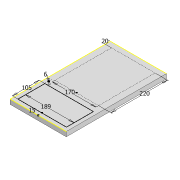
# Autodesk Inventor part: Platform
Saved by Autodesk Inventor 2020 (Build 240168000, 168)
## iProperties
Created: 2021-06-25
Part Number: Platform
Material: Generic
Document SubType Name: Modeling
Designer: Aidan Lee
Density: 1 g/cm^3
Appearance: Default
Author: Aidan Lee
Autodesk Inventor part; units mm, degrees
ref_plane "YZ Plane" through (0, 0, 0) normal (1, 0, 0) x (0, 1, 0)
ref_plane "XZ Plane" through (0, 0, 0) normal (0, 1, 0) x (-1, 0, 0)
ref_plane "XY Plane" through (0, 0, 0) normal (0, 0, 1) x (1, 0, 0)
sketch "Sketch1" plane through (0, 0, 0) normal (0, 0, 1) x (1, 0, 0)
  line L0 (0, 0) -> (219, 0)
  line L1 (219, 0) -> (219, 18)
  line L2 (219, 18) -> (0, 18)
  line L3 (0, 18) -> (0, 0)
  dimension "d0" = 18
  dimension "d1" = 219
  constraints: 8 end point, 2 parallel, 1 horizontal, 1 perpendicular
  measures "d0" distance of L2.end L0.start
  measures "d1" distance of L0.start L0.end
extrude "Extrusion1" add sketch "Sketch1" against normal blind 390
sketch "Sketch2" plane through (0, 18, 0) normal (0, 1, 0) x (1, 0, 0)
  line L0 (24.5, 150) -> (194.5, 150) construction
  line L1 (194.5, 150) -> (194.5, 370) construction
  line L2 (194.5, 370) -> (24.5, 370) construction
  line L3 (24.5, 370) -> (24.5, 150) construction
  line L4 (15, 15) -> (204, 15)
  line L5 (204, 15) -> (204, 120)
  line L6 (204, 120) -> (15, 120)
  line L7 (15, 120) -> (15, 15)
  line L8 (219, 0) -> (0, 0) projected
  line L9 (0, 0) -> (0, 390) projected
  line L10 (0, 390) -> (219, 390) projected
  circle A0 centre (15, 135) radius 3
  line L11 (15, 120) -> (15, 150) construction
  point P0 (109.5, 0)
  point P1 (109.5, 15)
  point P2 (109.5, 0)
  point P3 (109.5, 150)
  point P4 (15, 135)
  dimension "d4" = 220
  dimension "d5" = 170
  dimension "d6" = 189
  dimension "d7" = 105
  dimension "d9" = 15
  dimension "d11" = 20
  dimension "d12" = 6
  constraints: 18 end point, 5 midpoint, 4 parallel, 3 vertical alignment, 2 horizontal, 2 perpendicular, 1 centre point, 1 coincident, 1 horizontal alignment, 1 vertical
  measures "d4" distance of L0.end L1.end
  measures "d5" distance of L0.start L0.end
  measures "d6" distance of L4.start L4.end
  measures "d7" distance of L6.end L4.start
  measures "d9" distance between parallel lines of L8 L4
  measures "d11" distance between parallel lines of L10 L2
  measures "d12" diameter of A0
body "Solid1"
